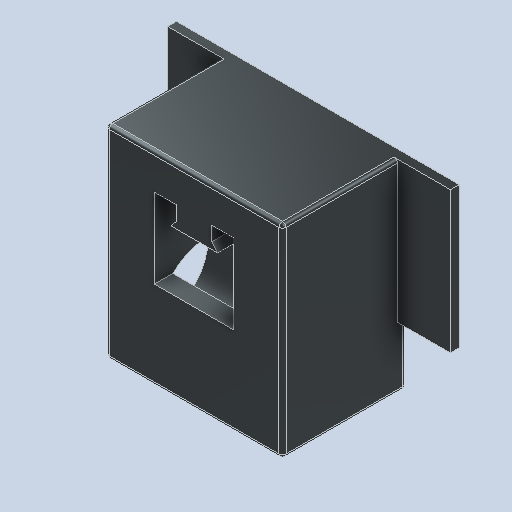
# Autodesk Inventor part: Motor_case
Saved by Autodesk Inventor 2025.2 (Build 292293000, 293)
## iProperties
Created: 2025-01-08
Part Number: Motor_case
Material: Iron, Ductile
Document SubType Name: Modeling
Designer: Sergio Quintero
Density: 7.15 g/cm^3
Appearance: Iron Gray
Author: Sergio Quintero
Autodesk Inventor part; units mm, degrees
ref_plane "YZ Plane" through (0, 0, 0) normal (1, 0, 0) x (0, 1, 0)
ref_plane "XZ Plane" through (0, 0, 0) normal (0, 1, 0) x (-1, 0, 0)
ref_plane "XY Plane" through (0, 0, 0) normal (0, 0, 1) x (1, 0, 0)
sketch "Sketch1" plane through (0, 0, 0) normal (0, 0, 1) x (1, 0, 0)
  line L0 (-50, -57.5) -> (50, -57.5)
  line L1 (50, -57.5) -> (50, 57.5)
  line L2 (50, 57.5) -> (-50, 57.5)
  line L3 (-50, 57.5) -> (-50, -57.5)
  line L4 (-50, -57.5) -> (50, 57.5) construction
  line L5 (50, -57.5) -> (-50, 57.5) construction
  point P0 (0, 0)
  dimension "d0" = 100
  dimension "d1" = 115
  constraints: 12 end point, 2 midpoint, 2 parallel, 1 horizontal, 1 perpendicular
  measures "d0" distance of L2.end L1.end
  measures "d1" distance of L1.end L0.end
extrude "Extrusion1" add sketch "Sketch1" along normal blind 70
sketch "Sketch2" plane through (50, -57.5, 0) normal (1, 0, 0) x (0, 0, -1)
  line L0 (0, 0) -> (0, 115) projected
  line L1 (0, 115) -> (-5, 115)
  line L2 (-5, 115) -> (-5, 35)
  line L3 (-5, 35) -> (0, 35)
  line L4 (0, 35) -> (0, 115)
  point P0 (0, 57.5)
  point P1 (0, 35)
  dimension "d4" = 5
  dimension "d5" = 80
  constraints: 8 end point, 2 parallel, 1 horizontal, 1 perpendicular
  measures "d4" distance of L3.end L2.end
  measures "d5" distance of L2.end L1.end
extrude "Extrusion2" add sketch "Sketch2" along normal blind 30
mirror "Mirror1" about plane through (0, 0, 0) normal (1, 0, 0) of "Extrusion2"
sketch "Sketch3" plane through (0, 0, 70) normal (0, 0, 1) x (1, 0, 0)
  line L0 (-22.5, 37.5) -> (22.5, 37.5)
  line L1 (22.5, 37.5) -> (22.5, -7.5)
  line L2 (22.5, -7.5) -> (-22.5, -7.5)
  line L3 (-22.5, -7.5) -> (-22.5, 37.5)
  line L4 (0, 50) -> (0, -57.5) construction
  line L5 (-50, -57.5) -> (50, -57.5) construction
  line L6 (50, 57.5) -> (-50, 57.5) projected
  point P0 (0, 0)
  point P1 (22.5, 15)
  dimension "d8" = 45
  dimension "d9" = 45
  dimension "d10" = 20
  constraints: 10 end point, 2 midpoint, 2 parallel, 1 horizontal, 1 perpendicular, 2 other
  measures "d8" distance between parallel lines of L2 L0
  measures "d9" distance from line of point (22.5, 15) L3
extrude "Extrusion3" cut sketch "Sketch3" against normal through all
sketch "Sketch4" plane through (-50, -57.5, 70) normal (-1, 0, 0) x (0, 0, 1)
  circle A0 centre (-30, 30) radius 28
  line L0 (0, 115) -> (0, 0) projected
  line L1 (-70, 0) -> (0, 0) projected
  point P0 (-70, 57.5)
  dimension "d13" = 56
  dimension "d14" = 30
  dimension "d15" = 30
  constraints: 1 centre point
  measures "d13" diameter of A0
  measures "d14" distance from line of A0.centre L0
  measures "d15" distance from line of A0.centre L1
extrude "Extrusion4" cut sketch "Sketch4" against normal blind 80
sketch "Sketch5" plane through (0, 0, 70) normal (0, 0, 1) x (1, 0, 0)
  line L0 (-20, -2.5) -> (20, -2.5) projected
  line L1 (20, -2.5) -> (20, 37.5) projected
  line L2 (20, 37.5) -> (10, 37.5) projected
  line L3 (10, 37.5) -> (10, 29.5) projected
  line L4 (10, 29.5) -> (13.2139, 25.6698) projected
  line L5 (13.2139, 25.6698) -> (-13.2139, 25.6698) projected
  line L6 (-13.2139, 25.6698) -> (-10, 29.5) projected
  line L7 (-10, 29.5) -> (-10, 37.5) projected
  line L8 (-10, 37.5) -> (-20, 37.5) projected
  line L9 (-20, 37.5) -> (-20, -2.5) projected
  line L10 (10, 37.5) -> (-10, 37.5)
  line L11 (-22.5, 37.5) -> (22.5, 37.5) projected
  point P0 (0, 0)
  constraints: 2 end point, 1 collinear
extrude "Extrusion5" add sketch "Sketch5" against normal up to surface (70 mm away) contours L10 L3 L4 L5 L6 L7
fillet "Fillet1" radius 2 11 edges at (50, 0, 70) (0, -57.5, 70) (-50, 0, 70) (0, 57.5, 70) (50, -57.5, 35) (0, -57.5, 0) (50, -40, 0) (-50, -57.5, 35) (50, 57.5, 37.5) (-50, 57.5, 37.5) (-50, -40, 0)
body "Solid1"
